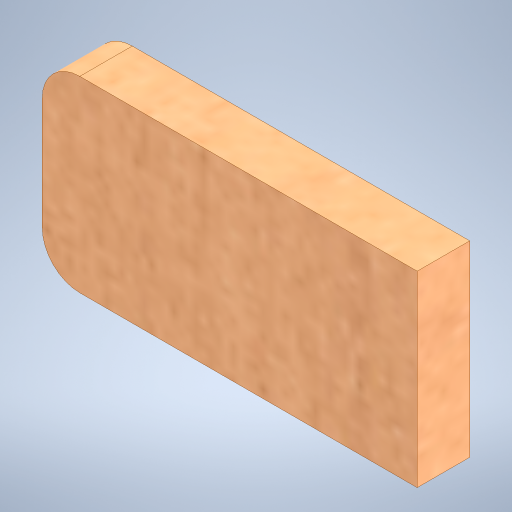
# Autodesk Inventor part: DedoV2
Saved by Autodesk Inventor 2023.1 (Build 271208000, 208)
## iProperties
Created: 2022-10-30
Part Number: DedoV2
Material: MDF Medium Density Fiberboard
Document SubType Name: Modeling
Designer: Daniel Peña
Density: 0.8 g/cm^3
Appearance: Cherry - Natural Low Gloss
Author: Daniel Peña
Autodesk Inventor part; units mm, degrees
ref_plane "YZ Plane" through (0, 0, 0) normal (1, 0, 0) x (0, 1, 0)
ref_plane "XZ Plane" through (0, 0, 0) normal (0, 1, 0) x (-1, 0, 0)
ref_plane "XY Plane" through (0, 0, 0) normal (0, 0, 1) x (1, 0, 0)
sketch "Sketch1" plane through (0, 0, 0) normal (0, 0, 1) x (1, 0, 0)
  line L0 (-14.3627, 11.329) -> (30.6373, 11.329)
  line L1 (30.6373, 11.329) -> (30.6373, -13.671)
  line L2 (30.6373, -13.671) -> (-14.3627, -13.671)
  line L3 (-19.3627, -8.671) -> (-19.3627, 6.329)
  arc A0 (-14.3627, 11.329) -> (-19.3627, 6.329) centre (-14.3627, 6.329) ccw
  arc A1 (-19.3627, -8.671) -> (-14.3627, -13.671) centre (-14.3627, -8.671) ccw
  point P0 (0, 0)
  point P1 (-19.3627, 11.329)
  point P2 (-19.3627, -13.671)
  dimension "d0" = 25
  dimension "d1" = 50
  dimension "d2" = 5
  constraints: 8 end point, 4 point on circle, 4 point on line, 4 tangent, 2 centre point, 2 parallel, 1 equal radius, 1 horizontal, 1 perpendicular
  measures "d0" distance of point (-19.363, -13.671) point (-19.363, 11.329)
  measures "d1" distance of point (-19.363, 11.329) L0.end
  measures "d2" radius of A0
extrude "Extrusion1" add sketch "Sketch1" along normal blind 7
body "Solid1"
